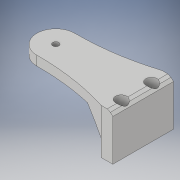
# Autodesk Inventor part: 000.403 - Верхний рычаг
Saved by Autodesk Inventor 2019 (Build 230136000, 136)
## iProperties
Created: 2020-04-03
Part Number: 000.403 - Верхний рычаг
Material: Типовые
Document SubType Name: Modeling
Designer: Петров Иван
Density: 1 g/cm^3
Appearance: По умолчанию
Author: Петров Иван
Autodesk Inventor part; units mm, degrees
ref_plane "YZ Plane" through (0, 0, 0) normal (1, 0, 0) x (0, 1, 0)
ref_plane "XZ Plane" through (0, 0, 0) normal (0, 1, 0) x (-1, 0, 0)
ref_plane "XY Plane" through (0, 0, 0) normal (0, 0, 1) x (1, 0, 0)
sketch "Эскиз1" plane through (0, 0, 0) normal (0, 1, 0) x (-1, 0, 0)
  circle A0 centre (0, 0) radius 1.6
  circle A1 centre (0, -0.0001) radius 5
  line L0 (-40, -6.3417) -> (-40, 6.3417)
  line L1 (-40, 16) -> (-46.0917, 16)
  line L2 (-46.0917, -16) -> (-40, -16)
  line L3 (-40, -16) -> (-40, -9.6583)
  line L4 (-40, -6.3417) -> (-40, -9.6583)
  line L5 (-40, 9.6583) -> (-40, 6.3417)
  line L6 (-40, 9.6583) -> (-40, 16)
  line L7 (-40, 16) -> (-46.0917, 16)
  line L8 (-46.0917, 16) -> (-46.0917, -16)
  line L9 (-46.0917, -16) -> (-40, -16)
  line L10 (-40, -16) -> (-40, 16)
  circle A2 centre (0, -0.0001) radius 10
  arc A3 (-40, 16) -> (-0.0411, 9.9998) centre (-0.586, 142.4269) ccw
  arc A4 (-0.0411, -10) -> (-40, -16) centre (-0.5865, -142.4271) ccw
  point P0 (0, 0)
  dimension "d0" = 20
  dimension "d1" = 132.4282
  dimension "d2" = 132.4282
  constraints: 22 end point, 6 point on circle, 5 centre point, 4 horizontal, 2 parallel, 1 coincident, 1 perpendicular, 1 tangent, 1 vertical, 1 other
  measures "d0" diameter of A2
  measures "d1" radius of A3
  measures "d2" radius of A4
extrude "Выдавливание1" add sketch "Эскиз1" along normal blind 5 contours A1 | L4 L3 L2 L8 L1 L6 L5 L0 | L0 L5 L6 A3 A2 A4 L3 L4 | A2
sketch "Эскиз2" plane through (0, 0, 0) normal (0, -1, 0) x (1, 0, 0)
  circle A0 centre (42.5, -8) radius 1.25 projected
  circle A1 centre (0, 0) radius 1.6 projected
  line L0 (46.0917, -16) -> (40, -16) projected
  line L1 (46.0917, 16) -> (46.0917, -16) projected
  line L2 (40, 16) -> (46.0917, 16) projected
  arc A2 (0.0411, 9.9998) -> (40, 16) centre (0.586, 142.4269) ccw projected
  arc A3 (0.0411, 9.9998) -> (0.0411, -10) centre (0, -0.0001) ccw projected
  arc A4 (40, -16) -> (0.0411, -10) centre (0.5865, -142.4271) ccw projected
  circle A5 centre (42.5, 8) radius 1.25 projected
  point P0 (0, 0)
extrude "Выдавливание2" cut sketch "Эскиз2" against normal blind 5 contours A0 | A5
sketch "Эскиз3" plane through (0, 0, 0) normal (0, -1, 0) x (1, 0, 0)
  line L0 (46.0917, 16) -> (46.0917, -16) projected
  arc A0 (40, -16) -> (0.0411, -10) centre (0.5865, -142.4271) ccw projected
  line L1 (46.0917, 16) -> (40, 16)
  line L2 (40, 16) -> (40, -16)
  line L3 (40, -16) -> (46.0917, -16)
  line L4 (46.0917, -16) -> (46.0917, 16)
  circle A1 centre (42.5, 8) radius 1.25 projected
  circle A2 centre (42.5, 8) radius 1.25
  circle A3 centre (42.5, -8) radius 1.25 projected
  circle A4 centre (42.5, -8) radius 1.25
  point P0 (0, 0)
  constraints: 8 end point, 2 centre point, 2 coincident, 2 parallel, 1 horizontal, 1 perpendicular
extrude "Выдавливание3" add sketch "Эскиз3" along normal blind 18.8
chamfer "Фаска1" distance 10 angle 45 1 edges at (40, 0, 0)
sketch "Эскиз4" plane through (0, 5, 0) normal (0, 1, 0) x (1, 0, 0)
  circle A0 centre (42.5, -8) radius 1.25 projected
  circle A1 centre (42.5, -8) radius 3
  circle A2 centre (42.5, 8) radius 1.25 projected
  circle A3 centre (42.5, 8) radius 3
  point P0 (0, 0)
  dimension "d12" = 6
  dimension "d13" = 6
  constraints: 2 centre point, 2 coincident
  measures "d12" diameter of A1
  measures "d13" diameter of A3
extrude "Выдавливание4" cut sketch "Эскиз4" against normal blind 20
chamfer "Фаска2" distance 2 angle 45 1 edges at (46.0917, 5, 0)
chamfer "Фаска3" distance 1 angle 45 3 edges at (44.0917, 5, 0) (44.0917, 5, 13.2715) (44.0917, 5, -13.2715)
equation "\"d2\" = d1"
